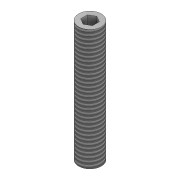
# Autodesk Inventor part: Tornillo Gusano Allen M3x16mm
Saved by Autodesk Inventor 2020.3 (Build 243373000, 373)
## iProperties
Created: 2020-05-17
Part Number: Tornillo Gusano Allen M3x16mm
Material: Genérico
Document SubType Name: Modeling
Designer: Pipi
Density: 1 g/cm^3
Appearance: Goma - Negro - Versión 1.1
Author: Pipi
Autodesk Inventor part; units mm, degrees
ref_plane "YZ Plane" through (0, 0, 0) normal (1, 0, 0) x (0, 1, 0)
ref_plane "XZ Plane" through (0, 0, 0) normal (0, 1, 0) x (-1, 0, 0)
ref_plane "XY Plane" through (0, 0, 0) normal (0, 0, 1) x (1, 0, 0)
sketch "Boceto1" plane through (0, 0, 0) normal (0, 1, 0) x (-1, 0, 0)
  circle A0 centre (5.4687, 11.9791) radius 1.5
  point P0 (0, 0)
  dimension "d0" = 3
  constraints: 1 centre point
  measures "d0" diameter of A0
extrude "Extrusión1" add sketch "Boceto1" along normal blind 16
thread "Rosca1" size "M3x0.5" class "6g" standard "ANSI Metric M Profile" length 430
sketch "Boceto2" plane through (-5.4687, 16, 11.9791) normal (0, 1, 0) x (1, 0, 0)
  line L0 (0, 0.9122) -> (0.79, 0.4561)
  line L1 (0.79, 0.4561) -> (0.79, -0.4561)
  line L2 (0.79, -0.4561) -> (0, -0.9122)
  line L3 (0, -0.9122) -> (-0.79, -0.4561)
  line L4 (-0.79, -0.4561) -> (-0.79, 0.4561)
  line L5 (-0.79, 0.4561) -> (0, 0.9122)
  point P0 (5.4687, 11.9791)
  point P1 (0, 0)
  dimension "d5" = 1.58
  constraints: 12 end point, 13 other
  measures "d5" distance between parallel lines of L2 L5
extrude "Extrusión2" cut sketch "Boceto2" against normal blind 1.2
